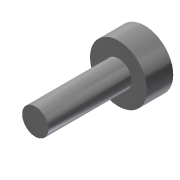
# Autodesk Inventor part: ThumbScrew
Saved by Autodesk Inventor 2014 (Build 180170000, 170)
## iProperties
Created: 2014-09-17
Part Number: ThumbScrew
Material: Generic
Document SubType Name: Modeling
Designer: Peele
Density: 1 g/cm^3
Appearance: Galvanized
Author: Peele
Autodesk Inventor part; units mm, degrees
ref_plane "YZ Plane" through (0, 0, 0) normal (1, 0, 0) x (0, 1, 0)
ref_plane "XZ Plane" through (0, 0, 0) normal (0, 1, 0) x (-1, 0, 0)
ref_plane "XY Plane" through (0, 0, 0) normal (0, 0, 1) x (1, 0, 0)
sketch "Sketch1" plane through (0, 0, 0) normal (0, 0, 1) x (1, 0, 0)
  line L0 (0, 0) -> (6.5, 0)
  line L1 (6.5, 0) -> (6.5, -6)
  line L2 (6.5, -6) -> (3, -6)
  line L3 (3, -6) -> (3, -25)
  line L4 (3, -25) -> (0, -25)
  line L5 (0, -25) -> (0, 0)
  dimension "d0" = 6.5
  dimension "d1" = 3
  dimension "d2" = 6
  dimension "d3" = 19
  constraints: 12 end point, 3 parallel, 1 horizontal, 1 perpendicular, 1 vertical
  measures "d0" distance between parallel lines of L5 L1
  measures "d1" distance between parallel lines of L5 L3
  measures "d2" distance of L0.end L1.end
  measures "d3" distance of L2.end L3.end
revolve "Revolution1" add sketch "Sketch1" angle 360 about axis through (0, -25, 0) along (0, 1, 0)
body "Solid1"
